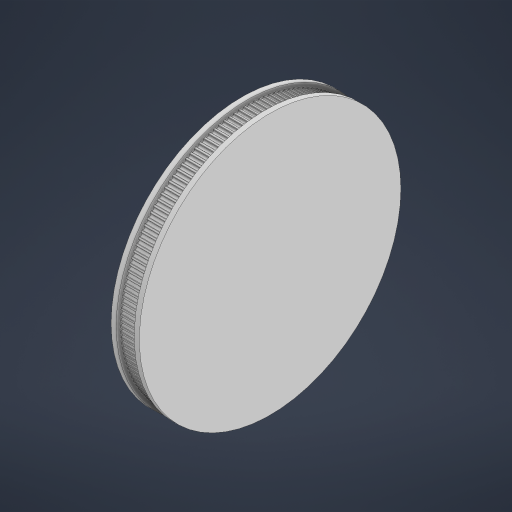
# Autodesk Inventor part: GT2 Pulley
Saved by Autodesk Inventor 2024 (Build 280153000, 153)
## iProperties
Created: 2023-10-25
Part Number: GT2 Pulley
Material: Generic
Document SubType Name: Modeling
Designer: avsar
Density: 1 g/cm^3
Appearance: Default
Author: avsar
Autodesk Inventor part; units mm, degrees
ref_plane "YZ Plane" through (0, 0, 0) normal (1, 0, 0) x (0, 1, 0)
ref_plane "XZ Plane" through (0, 0, 0) normal (0, 1, 0) x (-1, 0, 0)
ref_plane "XY Plane" through (0, 0, 0) normal (0, 0, 1) x (1, 0, 0)
sketch "Sketch1" plane through (0, 0, 0) normal (1, 0, 0) x (0, 1, 0)
  circle A0 centre (0, 0) radius 49.4023 construction
  circle A1 centre (0, 0) radius 48.6523 construction
  line L0 (0, 0) -> (49.4023, 0) construction
  line L1 (0, 0) -> (0, -49.4023) construction
  circle A2 centre (49.2073, 0) radius 0.555 construction
  line L2 (0, 0) -> (49.3623, -1.9892) construction
  circle A3 centre (49.1674, -1.9814) radius 0.555 construction
  circle A4 centre (49.2473, -0.7039) radius 0.15 construction
  circle A5 centre (49.2357, -1.2797) radius 0.15 construction
  arc A6 (48.6523, 0) -> (49.2388, -0.5541) centre (49.2073, 0) ccw
  arc A7 (49.3973, -0.706) -> (49.2388, -0.5541) centre (49.2473, -0.7039) ccw
  arc A8 (49.3857, -1.2836) -> (49.3973, -0.706) centre (0, 0) ccw
  arc A9 (49.2212, -1.429) -> (49.3857, -1.2836) centre (49.2357, -1.2797) ccw
  arc A10 (49.2212, -1.429) -> (48.6129, -1.959) centre (49.1674, -1.9814) ccw
  arc A11 (48.6129, -1.959) -> (48.6523, 0) centre (0, 0) ccw
  dimension "d0" = 98.8047
  dimension "d1" = -0.75
  dimension "d2" = 1.11
  dimension "d4" = 87.692
  dimension "d5" = 0.3
  constraints: 25 point on circle, 12 centre point, 8 equal radius, 8 tangent, 6 end point, 4 point on line, 1 coincident, 1 concentric, 1 horizontal, 1 perpendicular
  measures "d0" diameter of A0
  measures "d1" radial gap between concentric circles of A0 A1
  measures "d2" diameter of A2
  measures "d4" angle of L1 L2
  measures "d5" diameter of A4
extrude "Extrusion1" add sketch "Sketch1" along normal mid plane 7
pattern_circular "Circular Pattern1" count 156 over 360 about axis through (-10, 0, 0) along (1, 0, 0) of "Extrusion1"
sketch "Sketch2" plane through (0, 0, 0) normal (1, 0, 0) x (0, 1, 0)
  arc A0 (48.6129, 1.959) -> (49.2212, 1.429) centre (49.1674, 1.9814) ccw projected
  circle A1 centre (0, 0) radius 48.6523
  constraints: 1 coincident, 3 other
extrude "Extrusion2" add sketch "Sketch2" along normal mid plane 7
sketch "Sketch3" plane through (3.5, 0, 0) normal (1, 0, 0) x (0, 0, -1)
  circle A0 centre (0, 0) radius 51
  dimension "d13" = 102
  constraints: 1 centre point, 1 coincident
  measures "d13" diameter of A0
extrude "Extrusion3" add sketch "Sketch3" along normal blind 2
sketch "Sketch4" plane through (-3.5, 0, 0) normal (-1, 0, 0) x (0, 0, 1)
  circle A0 centre (0, 0) radius 51 projected
extrude "Extrusion4" add sketch "Sketch4" along normal blind 2
equation "\"d0\" = OD_"
equation "\"d1\" = H_"
equation "\"d2\" = BTD_"
equation "\"d4\" = TH_"
equation "\"d5\" = PTR_"
equation "\"d6\" = EX_"
equation "\"d11\" = EX_"
equation "\"U_\" = 0.254"
equation "\"H_\" = -0.75"
equation "\"P_\" = 2"
equation "\"BTD_\" = 1.11"
equation "\"PTR_\" = 0.3"
equation "\"EX_\" = 7"
equation "\"OD_\" = PD_ - 2 * U_"
equation "\"TH_\" = 87.692308deg"
equation "\"PD_\" = 99.312684"
body "Solid1"
